Autodesk Inventor part; units mm, degrees
(part 11 of 15)
  arc A4843 (8.9412, 10.184) -> (9.0428, 10.184) centre (8.992, 10.184) ccw
  line L2248 (8.992, 12.216) -> (10.008, 12.216)
  arc A4844 (10.008, 12.1652) -> (10.008, 12.2668) centre (10.008, 12.216) ccw
  arc A4845 (8.992, 12.2668) -> (8.992, 12.1652) centre (8.992, 12.216) ccw
  line L2249 (10.008, 12.216) -> (10.008, 10.184)
  arc A4846 (9.9572, 10.184) -> (10.0588, 10.184) centre (10.008, 10.184) ccw
  arc A4847 (10.0588, 12.216) -> (9.9572, 12.216) centre (10.008, 12.216) ccw
  line L2250 (10.008, 10.184) -> (8.992, 10.184)
  arc A4848 (8.992, 10.2348) -> (8.992, 10.1332) centre (8.992, 10.184) ccw
  arc A4849 (10.008, 10.1332) -> (10.008, 10.2348) centre (10.008, 10.184) ccw
  line L2251 (1.008, 14.216) -> (1.008, 12.184)
  arc A4850 (0.9572, 12.184) -> (1.0588, 12.184) centre (1.008, 12.184) ccw
  arc A4851 (1.0588, 14.216) -> (0.9572, 14.216) centre (1.008, 14.216) ccw
  line L2252 (1.008, 12.184) -> (-0.008, 12.184)
  arc A4852 (-0.008, 12.2348) -> (-0.008, 12.1332) centre (-0.008, 12.184) ccw
  arc A4853 (1.008, 12.1332) -> (1.008, 12.2348) centre (1.008, 12.184) ccw
  line L2253 (-0.008, 12.184) -> (-0.008, 14.216)
  arc A4854 (0.0428, 14.216) -> (-0.0588, 14.216) centre (-0.008, 14.216) ccw
  arc A4855 (-0.0588, 12.184) -> (0.0428, 12.184) centre (-0.008, 12.184) ccw
  line L2254 (-0.008, 14.216) -> (1.008, 14.216)
  arc A4856 (1.008, 14.1652) -> (1.008, 14.2668) centre (1.008, 14.216) ccw
  arc A4857 (-0.008, 14.2668) -> (-0.008, 14.1652) centre (-0.008, 14.216) ccw
  line L2255 (-6.016, 13.208) -> (-3.984, 13.208)
  arc A4858 (-3.984, 13.1572) -> (-3.984, 13.2588) centre (-3.984, 13.208) ccw
  arc A4859 (-6.016, 13.2588) -> (-6.016, 13.1572) centre (-6.016, 13.208) ccw
  line L2256 (-3.984, 13.208) -> (-3.984, 12.192)
  arc A4860 (-4.0348, 12.192) -> (-3.9332, 12.192) centre (-3.984, 12.192) ccw
  arc A4861 (-3.9332, 13.208) -> (-4.0348, 13.208) centre (-3.984, 13.208) ccw
  line L2257 (-3.984, 12.192) -> (-6.016, 12.192)
  arc A4862 (-6.016, 12.2428) -> (-6.016, 12.1412) centre (-6.016, 12.192) ccw
  arc A4863 (-3.984, 12.1412) -> (-3.984, 12.2428) centre (-3.984, 12.192) ccw
  line L2258 (-6.016, 12.192) -> (-6.016, 13.208)
  arc A4864 (-5.9652, 13.208) -> (-6.0668, 13.208) centre (-6.016, 13.208) ccw
  arc A4865 (-6.0668, 12.192) -> (-5.9652, 12.192) centre (-6.016, 12.192) ccw
  line L2259 (-6.016, 12.208) -> (-3.984, 12.208)
  arc A4866 (-3.984, 12.1572) -> (-3.984, 12.2588) centre (-3.984, 12.208) ccw
  arc A4867 (-6.016, 12.2588) -> (-6.016, 12.1572) centre (-6.016, 12.208) ccw
  line L2260 (-3.984, 12.208) -> (-3.984, 11.192)
  arc A4868 (-4.0348, 11.192) -> (-3.9332, 11.192) centre (-3.984, 11.192) ccw
  arc A4869 (-3.9332, 12.208) -> (-4.0348, 12.208) centre (-3.984, 12.208) ccw
  line L2261 (-3.984, 11.192) -> (-6.016, 11.192)
  arc A4870 (-6.016, 11.2428) -> (-6.016, 11.1412) centre (-6.016, 11.192) ccw
  arc A4871 (-3.984, 11.1412) -> (-3.984, 11.2428) centre (-3.984, 11.192) ccw
  line L2262 (-6.016, 11.192) -> (-6.016, 12.208)
  arc A4872 (-5.9652, 12.208) -> (-6.0668, 12.208) centre (-6.016, 12.208) ccw
  arc A4873 (-6.0668, 11.192) -> (-5.9652, 11.192) centre (-6.016, 11.192) ccw
  line L2263 (1.992, -2.816) -> (1.992, -0.784)
  arc A4874 (2.0428, -0.784) -> (1.9412, -0.784) centre (1.992, -0.784) ccw
  arc A4875 (1.9412, -2.816) -> (2.0428, -2.816) centre (1.992, -2.816) ccw
  line L2264 (1.992, -0.784) -> (3.008, -0.784)
  arc A4876 (3.008, -0.8348) -> (3.008, -0.7332) centre (3.008, -0.784) ccw
  arc A4877 (1.992, -0.7332) -> (1.992, -0.8348) centre (1.992, -0.784) ccw
  line L2265 (3.008, -0.784) -> (3.008, -2.816)
  arc A4878 (2.9572, -2.816) -> (3.0588, -2.816) centre (3.008, -2.816) ccw
  arc A4879 (3.0588, -0.784) -> (2.9572, -0.784) centre (3.008, -0.784) ccw
  line L2266 (3.008, -2.816) -> (1.992, -2.816)
  arc A4880 (1.992, -2.7652) -> (1.992, -2.8668) centre (1.992, -2.816) ccw
  arc A4881 (3.008, -2.8668) -> (3.008, -2.7652) centre (3.008, -2.816) ccw
  line L2267 (18.716, 12.192) -> (16.684, 12.192)
  arc A4882 (16.684, 12.2428) -> (16.684, 12.1412) centre (16.684, 12.192) ccw
  arc A4883 (18.716, 12.1412) -> (18.716, 12.2428) centre (18.716, 12.192) ccw
  line L2268 (16.684, 12.192) -> (16.684, 13.208)
  arc A4884 (16.7348, 13.208) -> (16.6332, 13.208) centre (16.684, 13.208) ccw
  arc A4885 (16.6332, 12.192) -> (16.7348, 12.192) centre (16.684, 12.192) ccw
  line L2269 (16.684, 13.208) -> (18.716, 13.208)
  arc A4886 (18.716, 13.1572) -> (18.716, 13.2588) centre (18.716, 13.208) ccw
  arc A4887 (16.684, 13.2588) -> (16.684, 13.1572) centre (16.684, 13.208) ccw
  line L2270 (18.716, 13.208) -> (18.716, 12.192)
  arc A4888 (18.6652, 12.192) -> (18.7668, 12.192) centre (18.716, 12.192) ccw
  arc A4889 (18.7668, 13.208) -> (18.6652, 13.208) centre (18.716, 13.208) ccw
  line L2271 (22.916, 12.192) -> (20.884, 12.192)
  arc A4890 (20.884, 12.2428) -> (20.884, 12.1412) centre (20.884, 12.192) ccw
  arc A4891 (22.916, 12.1412) -> (22.916, 12.2428) centre (22.916, 12.192) ccw
  line L2272 (20.884, 12.192) -> (20.884, 13.208)
  arc A4892 (20.9348, 13.208) -> (20.8332, 13.208) centre (20.884, 13.208) ccw
  arc A4893 (20.8332, 12.192) -> (20.9348, 12.192) centre (20.884, 12.192) ccw
  line L2273 (20.884, 13.208) -> (22.916, 13.208)
  arc A4894 (22.916, 13.1572) -> (22.916, 13.2588) centre (22.916, 13.208) ccw
  arc A4895 (20.884, 13.2588) -> (20.884, 13.1572) centre (20.884, 13.208) ccw
  line L2274 (22.916, 13.208) -> (22.916, 12.192)
  arc A4896 (22.8652, 12.192) -> (22.9668, 12.192) centre (22.916, 12.192) ccw
  arc A4897 (22.9668, 13.208) -> (22.8652, 13.208) centre (22.916, 13.208) ccw
  line L2275 (18.716, 1.792) -> (16.684, 1.792)
  arc A4898 (16.684, 1.8428) -> (16.684, 1.7412) centre (16.684, 1.792) ccw
  arc A4899 (18.716, 1.7412) -> (18.716, 1.8428) centre (18.716, 1.792) ccw
  line L2276 (16.684, 1.792) -> (16.684, 2.808)
  arc A4900 (16.7348, 2.808) -> (16.6332, 2.808) centre (16.684, 2.808) ccw
  arc A4901 (16.6332, 1.792) -> (16.7348, 1.792) centre (16.684, 1.792) ccw
  line L2277 (16.684, 2.808) -> (18.716, 2.808)
  arc A4902 (18.716, 2.7572) -> (18.716, 2.8588) centre (18.716, 2.808) ccw
  arc A4903 (16.684, 2.8588) -> (16.684, 2.7572) centre (16.684, 2.808) ccw
  line L2278 (18.716, 2.808) -> (18.716, 1.792)
  arc A4904 (18.6652, 1.792) -> (18.7668, 1.792) centre (18.716, 1.792) ccw
  arc A4905 (18.7668, 2.808) -> (18.6652, 2.808) centre (18.716, 2.808) ccw
  line L2279 (22.916, 1.792) -> (20.884, 1.792)
  arc A4906 (20.884, 1.8428) -> (20.884, 1.7412) centre (20.884, 1.792) ccw
  arc A4907 (22.916, 1.7412) -> (22.916, 1.8428) centre (22.916, 1.792) ccw
  line L2280 (20.884, 1.792) -> (20.884, 2.808)
  arc A4908 (20.9348, 2.808) -> (20.8332, 2.808) centre (20.884, 2.808) ccw
  arc A4909 (20.8332, 1.792) -> (20.9348, 1.792) centre (20.884, 1.792) ccw
  line L2281 (20.884, 2.808) -> (22.916, 2.808)
  arc A4910 (22.916, 2.7572) -> (22.916, 2.8588) centre (22.916, 2.808) ccw
  arc A4911 (20.884, 2.8588) -> (20.884, 2.7572) centre (20.884, 2.808) ccw
  line L2282 (22.916, 2.808) -> (22.916, 1.792)
  arc A4912 (22.8652, 1.792) -> (22.9668, 1.792) centre (22.916, 1.792) ccw
  arc A4913 (22.9668, 2.808) -> (22.8652, 2.808) centre (22.916, 2.808) ccw
  line L2283 (18.716, -8.608) -> (16.684, -8.608)
  arc A4914 (16.684, -8.5572) -> (16.684, -8.6588) centre (16.684, -8.608) ccw
  arc A4915 (18.716, -8.6588) -> (18.716, -8.5572) centre (18.716, -8.608) ccw
  line L2284 (16.684, -8.608) -> (16.684, -7.592)
  arc A4916 (16.7348, -7.592) -> (16.6332, -7.592) centre (16.684, -7.592) ccw
  arc A4917 (16.6332, -8.608) -> (16.7348, -8.608) centre (16.684, -8.608) ccw
  line L2285 (16.684, -7.592) -> (18.716, -7.592)
  arc A4918 (18.716, -7.6428) -> (18.716, -7.5412) centre (18.716, -7.592) ccw
  arc A4919 (16.684, -7.5412) -> (16.684, -7.6428) centre (16.684, -7.592) ccw
  line L2286 (18.716, -7.592) -> (18.716, -8.608)
  arc A4920 (18.6652, -8.608) -> (18.7668, -8.608) centre (18.716, -8.608) ccw
  arc A4921 (18.7668, -7.592) -> (18.6652, -7.592) centre (18.716, -7.592) ccw
  line L2287 (22.916, -8.608) -> (20.884, -8.608)
  arc A4922 (20.884, -8.5572) -> (20.884, -8.6588) centre (20.884, -8.608) ccw
  arc A4923 (22.916, -8.6588) -> (22.916, -8.5572) centre (22.916, -8.608) ccw
  line L2288 (20.884, -8.608) -> (20.884, -7.592)
  arc A4924 (20.9348, -7.592) -> (20.8332, -7.592) centre (20.884, -7.592) ccw
  arc A4925 (20.8332, -8.608) -> (20.9348, -8.608) centre (20.884, -8.608) ccw
  line L2289 (20.884, -7.592) -> (22.916, -7.592)
  arc A4926 (22.916, -7.6428) -> (22.916, -7.5412) centre (22.916, -7.592) ccw
  arc A4927 (20.884, -7.5412) -> (20.884, -7.6428) centre (20.884, -7.592) ccw
  line L2290 (22.916, -7.592) -> (22.916, -8.608)
  arc A4928 (22.8652, -8.608) -> (22.9668, -8.608) centre (22.916, -8.608) ccw
  arc A4929 (22.9668, -7.592) -> (22.8652, -7.592) centre (22.916, -7.592) ccw
  line L2291 (18.716, -19.008) -> (16.684, -19.008)
  arc A4930 (16.684, -18.9572) -> (16.684, -19.0588) centre (16.684, -19.008) ccw
  arc A4931 (18.716, -19.0588) -> (18.716, -18.9572) centre (18.716, -19.008) ccw
  line L2292 (16.684, -19.008) -> (16.684, -17.992)
  arc A4932 (16.7348, -17.992) -> (16.6332, -17.992) centre (16.684, -17.992) ccw
  arc A4933 (16.6332, -19.008) -> (16.7348, -19.008) centre (16.684, -19.008) ccw
  line L2293 (16.684, -17.992) -> (18.716, -17.992)
  arc A4934 (18.716, -18.0428) -> (18.716, -17.9412) centre (18.716, -17.992) ccw
  arc A4935 (16.684, -17.9412) -> (16.684, -18.0428) centre (16.684, -17.992) ccw
  line L2294 (18.716, -17.992) -> (18.716, -19.008)
  arc A4936 (18.6652, -19.008) -> (18.7668, -19.008) centre (18.716, -19.008) ccw
  arc A4937 (18.7668, -17.992) -> (18.6652, -17.992) centre (18.716, -17.992) ccw
  line L2295 (22.916, -19.008) -> (20.884, -19.008)
  arc A4938 (20.884, -18.9572) -> (20.884, -19.0588) centre (20.884, -19.008) ccw
  arc A4939 (22.916, -19.0588) -> (22.916, -18.9572) centre (22.916, -19.008) ccw
  line L2296 (20.884, -19.008) -> (20.884, -17.992)
  arc A4940 (20.9348, -17.992) -> (20.8332, -17.992) centre (20.884, -17.992) ccw
  arc A4941 (20.8332, -19.008) -> (20.9348, -19.008) centre (20.884, -19.008) ccw
  line L2297 (20.884, -17.992) -> (22.916, -17.992)
  arc A4942 (22.916, -18.0428) -> (22.916, -17.9412) centre (22.916, -17.992) ccw
  arc A4943 (20.884, -17.9412) -> (20.884, -18.0428) centre (20.884, -17.992) ccw
  line L2298 (22.916, -17.992) -> (22.916, -19.008)
  arc A4944 (22.8652, -19.008) -> (22.9668, -19.008) centre (22.916, -19.008) ccw
  arc A4945 (22.9668, -17.992) -> (22.8652, -17.992) centre (22.916, -17.992) ccw
  line L2299 (-1.784, -14.108) -> (-3.816, -14.108)
  arc A4946 (-3.816, -14.0572) -> (-3.816, -14.1588) centre (-3.816, -14.108) ccw
  arc A4947 (-1.784, -14.1588) -> (-1.784, -14.0572) centre (-1.784, -14.108) ccw
  line L2300 (-3.816, -14.108) -> (-3.816, -13.092)
  arc A4948 (-3.7652, -13.092) -> (-3.8668, -13.092) centre (-3.816, -13.092) ccw
  arc A4949 (-3.8668, -14.108) -> (-3.7652, -14.108) centre (-3.816, -14.108) ccw
  line L2301 (-3.816, -13.092) -> (-1.784, -13.092)
  arc A4950 (-1.784, -13.1428) -> (-1.784, -13.0412) centre (-1.784, -13.092) ccw
  arc A4951 (-3.816, -13.0412) -> (-3.816, -13.1428) centre (-3.816, -13.092) ccw
  line L2302 (-1.784, -13.092) -> (-1.784, -14.108)
  arc A4952 (-1.8348, -14.108) -> (-1.7332, -14.108) centre (-1.784, -14.108) ccw
  arc A4953 (-1.7332, -13.092) -> (-1.8348, -13.092) centre (-1.784, -13.092) ccw
  line L2303 (-10.092, -20.084) -> (-10.092, -22.116)
  arc A4954 (-10.1428, -22.116) -> (-10.0412, -22.116) centre (-10.092, -22.116) ccw
  arc A4955 (-10.0412, -20.084) -> (-10.1428, -20.084) centre (-10.092, -20.084) ccw
  line L2304 (-10.092, -22.116) -> (-11.108, -22.116)
  arc A4956 (-11.108, -22.0652) -> (-11.108, -22.1668) centre (-11.108, -22.116) ccw
  arc A4957 (-10.092, -22.1668) -> (-10.092, -22.0652) centre (-10.092, -22.116) ccw
  line L2305 (-11.108, -22.116) -> (-11.108, -20.084)
  arc A4958 (-11.0572, -20.084) -> (-11.1588, -20.084) centre (-11.108, -20.084) ccw
  arc A4959 (-11.1588, -22.116) -> (-11.0572, -22.116) centre (-11.108, -22.116) ccw
  line L2306 (-11.108, -20.084) -> (-10.092, -20.084)
  arc A4960 (-10.092, -20.1348) -> (-10.092, -20.0332) centre (-10.092, -20.084) ccw
  arc A4961 (-11.108, -20.0332) -> (-11.108, -20.1348) centre (-11.108, -20.084) ccw
  line L2307 (-7.216, -23.092) -> (-5.184, -23.092)
  arc A4962 (-5.184, -23.1428) -> (-5.184, -23.0412) centre (-5.184, -23.092) ccw
  arc A4963 (-7.216, -23.0412) -> (-7.216, -23.1428) centre (-7.216, -23.092) ccw
  line L2308 (-5.184, -23.092) -> (-5.184, -24.108)
  arc A4964 (-5.2348, -24.108) -> (-5.1332, -24.108) centre (-5.184, -24.108) ccw
  arc A4965 (-5.1332, -23.092) -> (-5.2348, -23.092) centre (-5.184, -23.092) ccw
  line L2309 (-5.184, -24.108) -> (-7.216, -24.108)
  arc A4966 (-7.216, -24.0572) -> (-7.216, -24.1588) centre (-7.216, -24.108) ccw
  arc A4967 (-5.184, -24.1588) -> (-5.184, -24.0572) centre (-5.184, -24.108) ccw
  line L2310 (-7.216, -24.108) -> (-7.216, -23.092)
  arc A4968 (-7.1652, -23.092) -> (-7.2668, -23.092) centre (-7.216, -23.092) ccw
  arc A4969 (-7.2668, -24.108) -> (-7.1652, -24.108) centre (-7.216, -24.108) ccw
  line L2311 (-1.784, -18.108) -> (-3.816, -18.108)
  arc A4970 (-3.816, -18.0572) -> (-3.816, -18.1588) centre (-3.816, -18.108) ccw
  arc A4971 (-1.784, -18.1588) -> (-1.784, -18.0572) centre (-1.784, -18.108) ccw
  line L2312 (-3.816, -18.108) -> (-3.816, -17.092)
  arc A4972 (-3.7652, -17.092) -> (-3.8668, -17.092) centre (-3.816, -17.092) ccw
  arc A4973 (-3.8668, -18.108) -> (-3.7652, -18.108) centre (-3.816, -18.108) ccw
  line L2313 (-3.816, -17.092) -> (-1.784, -17.092)
  arc A4974 (-1.784, -17.1428) -> (-1.784, -17.0412) centre (-1.784, -17.092) ccw
  arc A4975 (-3.816, -17.0412) -> (-3.816, -17.1428) centre (-3.816, -17.092) ccw
  line L2314 (-1.784, -17.092) -> (-1.784, -18.108)
  arc A4976 (-1.8348, -18.108) -> (-1.7332, -18.108) centre (-1.784, -18.108) ccw
  arc A4977 (-1.7332, -17.092) -> (-1.8348, -17.092) centre (-1.784, -17.092) ccw
  line L2315 (-8.084, -21.108) -> (-10.116, -21.108)
  arc A4978 (-10.116, -21.0572) -> (-10.116, -21.1588) centre (-10.116, -21.108) ccw
  arc A4979 (-8.084, -21.1588) -> (-8.084, -21.0572) centre (-8.084, -21.108) ccw
  line L2316 (-10.116, -21.108) -> (-10.116, -20.092)
  arc A4980 (-10.0652, -20.092) -> (-10.1668, -20.092) centre (-10.116, -20.092) ccw
  arc A4981 (-10.1668, -21.108) -> (-10.0652, -21.108) centre (-10.116, -21.108) ccw
  line L2317 (-10.116, -20.092) -> (-8.084, -20.092)
  arc A4982 (-8.084, -20.1428) -> (-8.084, -20.0412) centre (-8.084, -20.092) ccw
  arc A4983 (-10.116, -20.0412) -> (-10.116, -20.1428) centre (-10.116, -20.092) ccw
  line L2318 (-8.084, -20.092) -> (-8.084, -21.108)
  arc A4984 (-8.1348, -21.108) -> (-8.0332, -21.108) centre (-8.084, -21.108) ccw
  arc A4985 (-8.0332, -20.092) -> (-8.1348, -20.092) centre (-8.084, -20.092) ccw
  line L2319 (-1.784, -20.108) -> (-3.816, -20.108)
  arc A4986 (-3.816, -20.0572) -> (-3.816, -20.1588) centre (-3.816, -20.108) ccw
  arc A4987 (-1.784, -20.1588) -> (-1.784, -20.0572) centre (-1.784, -20.108) ccw
  line L2320 (-3.816, -20.108) -> (-3.816, -19.092)
  arc A4988 (-3.7652, -19.092) -> (-3.8668, -19.092) centre (-3.816, -19.092) ccw
  arc A4989 (-3.8668, -20.108) -> (-3.7652, -20.108) centre (-3.816, -20.108) ccw
  line L2321 (-3.816, -19.092) -> (-1.784, -19.092)
  arc A4990 (-1.784, -19.1428) -> (-1.784, -19.0412) centre (-1.784, -19.092) ccw
  arc A4991 (-3.816, -19.0412) -> (-3.816, -19.1428) centre (-3.816, -19.092) ccw
  line L2322 (-1.784, -19.092) -> (-1.784, -20.108)
  arc A4992 (-1.8348, -20.108) -> (-1.7332, -20.108) centre (-1.784, -20.108) ccw
  arc A4993 (-1.7332, -19.092) -> (-1.8348, -19.092) centre (-1.784, -19.092) ccw
  line L2323 (5.716, -19.808) -> (3.684, -19.808)
  arc A4994 (3.684, -19.7572) -> (3.684, -19.8588) centre (3.684, -19.808) ccw
  arc A4995 (5.716, -19.8588) -> (5.716, -19.7572) centre (5.716, -19.808) ccw
  line L2324 (3.684, -19.808) -> (3.684, -18.792)
  arc A4996 (3.7348, -18.792) -> (3.6332, -18.792) centre (3.684, -18.792) ccw
  arc A4997 (3.6332, -19.808) -> (3.7348, -19.808) centre (3.684, -19.808) ccw
  line L2325 (3.684, -18.792) -> (5.716, -18.792)
  arc A4998 (5.716, -18.8428) -> (5.716, -18.7412) centre (5.716, -18.792) ccw
  arc A4999 (3.684, -18.7412) -> (3.684, -18.8428) centre (3.684, -18.792) ccw
  line L2326 (5.716, -18.792) -> (5.716, -19.808)
  arc A5000 (5.6652, -19.808) -> (5.7668, -19.808) centre (5.716, -19.808) ccw
  arc A5001 (5.7668, -18.792) -> (5.6652, -18.792) centre (5.716, -18.792) ccw
  line L2327 (5.084, -14.792) -> (7.116, -14.792)
  arc A5002 (7.116, -14.8428) -> (7.116, -14.7412) centre (7.116, -14.792) ccw
  arc A5003 (5.084, -14.7412) -> (5.084, -14.8428) centre (5.084, -14.792) ccw
  line L2328 (7.116, -14.792) -> (7.116, -15.808)
  arc A5004 (7.0652, -15.808) -> (7.1668, -15.808) centre (7.116, -15.808) ccw
  arc A5005 (7.1668, -14.792) -> (7.0652, -14.792) centre (7.116, -14.792) ccw
  line L2329 (7.116, -15.808) -> (5.084, -15.808)
  arc A5006 (5.084, -15.7572) -> (5.084, -15.8588) centre (5.084, -15.808) ccw
  arc A5007 (7.116, -15.8588) -> (7.116, -15.7572) centre (7.116, -15.808) ccw
  line L2330 (5.084, -15.808) -> (5.084, -14.792)
  arc A5008 (5.1348, -14.792) -> (5.0332, -14.792) centre (5.084, -14.792) ccw
  arc A5009 (5.0332, -15.808) -> (5.1348, -15.808) centre (5.084, -15.808) ccw
  line L2331 (0.884, -14.792) -> (2.916, -14.792)
  arc A5010 (2.916, -14.8428) -> (2.916, -14.7412) centre (2.916, -14.792) ccw
  arc A5011 (0.884, -14.7412) -> (0.884, -14.8428) centre (0.884, -14.792) ccw
  line L2332 (2.916, -14.792) -> (2.916, -15.808)
  arc A5012 (2.8652, -15.808) -> (2.9668, -15.808) centre (2.916, -15.808) ccw
  arc A5013 (2.9668, -14.792) -> (2.8652, -14.792) centre (2.916, -14.792) ccw
  line L2333 (2.916, -15.808) -> (0.884, -15.808)
  arc A5014 (0.884, -15.7572) -> (0.884, -15.8588) centre (0.884, -15.808) ccw
  arc A5015 (2.916, -15.8588) -> (2.916, -15.7572) centre (2.916, -15.808) ccw
  line L2334 (0.884, -15.808) -> (0.884, -14.792)
  arc A5016 (0.9348, -14.792) -> (0.8332, -14.792) centre (0.884, -14.792) ccw
  arc A5017 (0.8332, -15.808) -> (0.9348, -15.808) centre (0.884, -15.808) ccw
  line L2335 (-7.216, -15.092) -> (-5.184, -15.092)
  arc A5018 (-5.184, -15.1428) -> (-5.184, -15.0412) centre (-5.184, -15.092) ccw
  arc A5019 (-7.216, -15.0412) -> (-7.216, -15.1428) centre (-7.216, -15.092) ccw
  line L2336 (-5.184, -15.092) -> (-5.184, -16.108)
  arc A5020 (-5.2348, -16.108) -> (-5.1332, -16.108) centre (-5.184, -16.108) ccw
  arc A5021 (-5.1332, -15.092) -> (-5.2348, -15.092) centre (-5.184, -15.092) ccw
  line L2337 (-5.184, -16.108) -> (-7.216, -16.108)
  arc A5022 (-7.216, -16.0572) -> (-7.216, -16.1588) centre (-7.216, -16.108) ccw
  arc A5023 (-5.184, -16.1588) -> (-5.184, -16.0572) centre (-5.184, -16.108) ccw
  line L2338 (-7.216, -16.108) -> (-7.216, -15.092)
  arc A5024 (-7.1652, -15.092) -> (-7.2668, -15.092) centre (-7.216, -15.092) ccw
  arc A5025 (-7.2668, -16.108) -> (-7.1652, -16.108) centre (-7.216, -16.108) ccw
  line L2339 (-1.784, -21.108) -> (-3.816, -21.108)
  arc A5026 (-3.816, -21.0572) -> (-3.816, -21.1588) centre (-3.816, -21.108) ccw
  arc A5027 (-1.784, -21.1588) -> (-1.784, -21.0572) centre (-1.784, -21.108) ccw
  line L2340 (-3.816, -21.108) -> (-3.816, -20.092)
  arc A5028 (-3.7652, -20.092) -> (-3.8668, -20.092) centre (-3.816, -20.092) ccw
  arc A5029 (-3.8668, -21.108) -> (-3.7652, -21.108) centre (-3.816, -21.108) ccw
  line L2341 (-3.816, -20.092) -> (-1.784, -20.092)
  arc A5030 (-1.784, -20.1428) -> (-1.784, -20.0412) centre (-1.784, -20.092) ccw
  arc A5031 (-3.816, -20.0412) -> (-3.816, -20.1428) centre (-3.816, -20.092) ccw
  line L2342 (-1.784, -20.092) -> (-1.784, -21.108)
  arc A5032 (-1.8348, -21.108) -> (-1.7332, -21.108) centre (-1.784, -21.108) ccw
  arc A5033 (-1.7332, -20.092) -> (-1.8348, -20.092) centre (-1.784, -20.092) ccw
  line L2343 (-10.116, -23.092) -> (-8.084, -23.092)
  arc A5034 (-8.084, -23.1428) -> (-8.084, -23.0412) centre (-8.084, -23.092) ccw
  arc A5035 (-10.116, -23.0412) -> (-10.116, -23.1428) centre (-10.116, -23.092) ccw
  line L2344 (-8.084, -23.092) -> (-8.084, -24.108)
  arc A5036 (-8.1348, -24.108) -> (-8.0332, -24.108) centre (-8.084, -24.108) ccw
  arc A5037 (-8.0332, -23.092) -> (-8.1348, -23.092) centre (-8.084, -23.092) ccw
  line L2345 (-8.084, -24.108) -> (-10.116, -24.108)
  arc A5038 (-10.116, -24.0572) -> (-10.116, -24.1588) centre (-10.116, -24.108) ccw
  arc A5039 (-8.084, -24.1588) -> (-8.084, -24.0572) centre (-8.084, -24.108) ccw
  line L2346 (-10.116, -24.108) -> (-10.116, -23.092)
  arc A5040 (-10.0652, -23.092) -> (-10.1668, -23.092) centre (-10.116, -23.092) ccw
  arc A5041 (-10.1668, -24.108) -> (-10.0652, -24.108) centre (-10.116, -24.108) ccw
  line L2347 (-1.784, -25.108) -> (-3.816, -25.108)
  arc A5042 (-3.816, -25.0572) -> (-3.816, -25.1588) centre (-3.816, -25.108) ccw
  arc A5043 (-1.784, -25.1588) -> (-1.784, -25.0572) centre (-1.784, -25.108) ccw
  line L2348 (-3.816, -25.108) -> (-3.816, -24.092)
  arc A5044 (-3.7652, -24.092) -> (-3.8668, -24.092) centre (-3.816, -24.092) ccw
  arc A5045 (-3.8668, -25.108) -> (-3.7652, -25.108) centre (-3.816, -25.108) ccw
  line L2349 (-3.816, -24.092) -> (-1.784, -24.092)
  arc A5046 (-1.784, -24.1428) -> (-1.784, -24.0412) centre (-1.784, -24.092) ccw
  arc A5047 (-3.816, -24.0412) -> (-3.816, -24.1428) centre (-3.816, -24.092) ccw
  line L2350 (-1.784, -24.092) -> (-1.784, -25.108)
  arc A5048 (-1.8348, -25.108) -> (-1.7332, -25.108) centre (-1.784, -25.108) ccw
  arc A5049 (-1.7332, -24.092) -> (-1.8348, -24.092) centre (-1.784, -24.092) ccw
  line L2351 (7.892, -20.316) -> (7.892, -18.284)
  arc A5050 (7.9428, -18.284) -> (7.8412, -18.284) centre (7.892, -18.284) ccw
  arc A5051 (7.8412, -20.316) -> (7.9428, -20.316) centre (7.892, -20.316) ccw
  line L2352 (7.892, -18.284) -> (8.908, -18.284)
  arc A5052 (8.908, -18.3348) -> (8.908, -18.2332) centre (8.908, -18.284) ccw
  arc A5053 (7.892, -18.2332) -> (7.892, -18.3348) centre (7.892, -18.284) ccw
  line L2353 (8.908, -18.284) -> (8.908, -20.316)
  arc A5054 (8.8572, -20.316) -> (8.9588, -20.316) centre (8.908, -20.316) ccw
  arc A5055 (8.9588, -18.284) -> (8.8572, -18.284) centre (8.908, -18.284) ccw
  line L2354 (8.908, -20.316) -> (7.892, -20.316)
  arc A5056 (7.892, -20.2652) -> (7.892, -20.3668) centre (7.892, -20.316) ccw
  arc A5057 (8.908, -20.3668) -> (8.908, -20.2652) centre (8.908, -20.316) ccw
  line L2355 (10.892, -20.316) -> (10.892, -18.284)
  arc A5058 (10.9428, -18.284) -> (10.8412, -18.284) centre (10.892, -18.284) ccw
  arc A5059 (10.8412, -20.316) -> (10.9428, -20.316) centre (10.892, -20.316) ccw
  line L2356 (10.892, -18.284) -> (11.908, -18.284)
  arc A5060 (11.908, -18.3348) -> (11.908, -18.2332) centre (11.908, -18.284) ccw
  arc A5061 (10.892, -18.2332) -> (10.892, -18.3348) centre (10.892, -18.284) ccw
  line L2357 (11.908, -18.284) -> (11.908, -20.316)
  arc A5062 (11.8572, -20.316) -> (11.9588, -20.316) centre (11.908, -20.316) ccw
  arc A5063 (11.9588, -18.284) -> (11.8572, -18.284) centre (11.908, -18.284) ccw
  line L2358 (11.908, -20.316) -> (10.892, -20.316)
  arc A5064 (10.892, -20.2652) -> (10.892, -20.3668) centre (10.892, -20.316) ccw
  arc A5065 (11.908, -20.3668) -> (11.908, -20.2652) centre (11.908, -20.316) ccw
  line L2359 (5.684, -18.792) -> (7.716, -18.792)
  arc A5066 (7.716, -18.8428) -> (7.716, -18.7412) centre (7.716, -18.792) ccw
  arc A5067 (5.684, -18.7412) -> (5.684, -18.8428) centre (5.684, -18.792) ccw
  line L2360 (7.716, -18.792) -> (7.716, -19.808)
  arc A5068 (7.6652, -19.808) -> (7.7668, -19.808) centre (7.716, -19.808) ccw
  arc A5069 (7.7668, -18.792) -> (7.6652, -18.792) centre (7.716, -18.792) ccw
  line L2361 (7.716, -19.808) -> (5.684, -19.808)
  arc A5070 (5.684, -19.7572) -> (5.684, -19.8588) centre (5.684, -19.808) ccw
  arc A5071 (7.716, -19.8588) -> (7.716, -19.7572) centre (7.716, -19.808) ccw
  line L2362 (5.684, -19.808) -> (5.684, -18.792)
  arc A5072 (5.7348, -18.792) -> (5.6332, -18.792) centre (5.684, -18.792) ccw
  arc A5073 (5.6332, -19.808) -> (5.7348, -19.808) centre (5.684, -19.808) ccw
  line L2363 (-10.116, -22.092) -> (-8.084, -22.092)
  arc A5074 (-8.084, -22.1428) -> (-8.084, -22.0412) centre (-8.084, -22.092) ccw
  arc A5075 (-10.116, -22.0412) -> (-10.116, -22.1428) centre (-10.116, -22.092) ccw
  line L2364 (-8.084, -22.092) -> (-8.084, -23.108)
  arc A5076 (-8.1348, -23.108) -> (-8.0332, -23.108) centre (-8.084, -23.108) ccw
  arc A5077 (-8.0332, -22.092) -> (-8.1348, -22.092) centre (-8.084, -22.092) ccw
  line L2365 (-8.084, -23.108) -> (-10.116, -23.108)
  arc A5078 (-10.116, -23.0572) -> (-10.116, -23.1588) centre (-10.116, -23.108) ccw
  arc A5079 (-8.084, -23.1588) -> (-8.084, -23.0572) centre (-8.084, -23.108) ccw
  line L2366 (-10.116, -23.108) -> (-10.116, -22.092)
  arc A5080 (-10.0652, -22.092) -> (-10.1668, -22.092) centre (-10.116, -22.092) ccw
  arc A5081 (-10.1668, -23.108) -> (-10.0652, -23.108) centre (-10.116, -23.108) ccw
  line L2367 (-10.116, -21.092) -> (-8.084, -21.092)
  arc A5082 (-8.084, -21.1428) -> (-8.084, -21.0412) centre (-8.084, -21.092) ccw
  arc A5083 (-10.116, -21.0412) -> (-10.116, -21.1428) centre (-10.116, -21.092) ccw
  line L2368 (-8.084, -21.092) -> (-8.084, -22.108)
  arc A5084 (-8.1348, -22.108) -> (-8.0332, -22.108) centre (-8.084, -22.108) ccw
  arc A5085 (-8.0332, -21.092) -> (-8.1348, -21.092) centre (-8.084, -21.092) ccw
  line L2369 (-8.084, -22.108) -> (-10.116, -22.108)
  arc A5086 (-10.116, -22.0572) -> (-10.116, -22.1588) centre (-10.116, -22.108) ccw
  arc A5087 (-8.084, -22.1588) -> (-8.084, -22.0572) centre (-8.084, -22.108) ccw
  line L2370 (-10.116, -22.108) -> (-10.116, -21.092)
  arc A5088 (-10.0652, -21.092) -> (-10.1668, -21.092) centre (-10.116, -21.092) ccw
  arc A5089 (-10.1668, -22.108) -> (-10.0652, -22.108) centre (-10.116, -22.108) ccw
  line L2371 (-19.116, 45.008) -> (-17.084, 45.008)
  arc A5090 (-17.084, 44.9572) -> (-17.084, 45.0588) centre (-17.084, 45.008) ccw
  arc A5091 (-19.116, 45.0588) -> (-19.116, 44.9572) centre (-19.116, 45.008) ccw
  line L2372 (-17.084, 45.008) -> (-17.084, 43.992)
  arc A5092 (-17.1348, 43.992) -> (-17.0332, 43.992) centre (-17.084, 43.992) ccw
  arc A5093 (-17.0332, 45.008) -> (-17.1348, 45.008) centre (-17.084, 45.008) ccw
  line L2373 (-17.084, 43.992) -> (-19.116, 43.992)
  arc A5094 (-19.116, 44.0428) -> (-19.116, 43.9412) centre (-19.116, 43.992) ccw
  arc A5095 (-17.084, 43.9412) -> (-17.084, 44.0428) centre (-17.084, 43.992) ccw
  line L2374 (-19.116, 43.992) -> (-19.116, 45.008)
  arc A5096 (-19.0652, 45.008) -> (-19.1668, 45.008) centre (-19.116, 45.008) ccw
  arc A5097 (-19.1668, 43.992) -> (-19.0652, 43.992) centre (-19.116, 43.992) ccw
  line L2375 (-19.116, 46.008) -> (-17.084, 46.008)
  arc A5098 (-17.084, 45.9572) -> (-17.084, 46.0588) centre (-17.084, 46.008) ccw
  arc A5099 (-19.116, 46.0588) -> (-19.116, 45.9572) centre (-19.116, 46.008) ccw
  line L2376 (-17.084, 46.008) -> (-17.084, 44.992)
  arc A5100 (-17.1348, 44.992) -> (-17.0332, 44.992) centre (-17.084, 44.992) ccw
  arc A5101 (-17.0332, 46.008) -> (-17.1348, 46.008) centre (-17.084, 46.008) ccw
  line L2377 (-17.084, 44.992) -> (-19.116, 44.992)
  arc A5102 (-19.116, 45.0428) -> (-19.116, 44.9412) centre (-19.116, 44.992) ccw
  arc A5103 (-17.084, 44.9412) -> (-17.084, 45.0428) centre (-17.084, 44.992) ccw
  line L2378 (-19.116, 44.992) -> (-19.116, 46.008)
  arc A5104 (-19.0652, 46.008) -> (-19.1668, 46.008) centre (-19.116, 46.008) ccw
  arc A5105 (-19.1668, 44.992) -> (-19.0652, 44.992) centre (-19.116, 44.992) ccw
  line L2379 (-23.284, 38.992) -> (-25.316, 38.992)
  arc A5106 (-25.316, 39.0428) -> (-25.316, 38.9412) centre (-25.316, 38.992) ccw
  arc A5107 (-23.284, 38.9412) -> (-23.284, 39.0428) centre (-23.284, 38.992) ccw
  line L2380 (-25.316, 38.992) -> (-25.316, 40.008)
  arc A5108 (-25.2652, 40.008) -> (-25.3668, 40.008) centre (-25.316, 40.008) ccw
  arc A5109 (-25.3668, 38.992) -> (-25.2652, 38.992) centre (-25.316, 38.992) ccw
  line L2381 (-25.316, 40.008) -> (-23.284, 40.008)
  arc A5110 (-23.284, 39.9572) -> (-23.284, 40.0588) centre (-23.284, 40.008) ccw
  arc A5111 (-25.316, 40.0588) -> (-25.316, 39.9572) centre (-25.316, 40.008) ccw
  line L2382 (-23.284, 40.008) -> (-23.284, 38.992)
  arc A5112 (-23.3348, 38.992) -> (-23.2332, 38.992) centre (-23.284, 38.992) ccw
  arc A5113 (-23.2332, 40.008) -> (-23.3348, 40.008) centre (-23.284, 40.008) ccw
  line L2383 (-22.016, 51.108) -> (-19.984, 51.108)
  arc A5114 (-19.984, 51.0572) -> (-19.984, 51.1588) centre (-19.984, 51.108) ccw
  arc A5115 (-22.016, 51.1588) -> (-22.016, 51.0572) centre (-22.016, 51.108) ccw
  line L2384 (-19.984, 51.108) -> (-19.984, 50.092)
  arc A5116 (-20.0348, 50.092) -> (-19.9332, 50.092) centre (-19.984, 50.092) ccw
  arc A5117 (-19.9332, 51.108) -> (-20.0348, 51.108) centre (-19.984, 51.108) ccw
  line L2385 (-19.984, 50.092) -> (-22.016, 50.092)
  arc A5118 (-22.016, 50.1428) -> (-22.016, 50.0412) centre (-22.016, 50.092) ccw
  arc A5119 (-19.984, 50.0412) -> (-19.984, 50.1428) centre (-19.984, 50.092) ccw
  line L2386 (-22.016, 50.092) -> (-22.016, 51.108)
  arc A5120 (-21.9652, 51.108) -> (-22.0668, 51.108) centre (-22.016, 51.108) ccw
  arc A5121 (-22.0668, 50.092) -> (-21.9652, 50.092) centre (-22.016, 50.092) ccw
  line L2387 (-19.984, 48.092) -> (-22.016, 48.092)
  arc A5122 (-22.016, 48.1428) -> (-22.016, 48.0412) centre (-22.016, 48.092) ccw
  arc A5123 (-19.984, 48.0412) -> (-19.984, 48.1428) centre (-19.984, 48.092) ccw
  line L2388 (-22.016, 48.092) -> (-22.016, 49.108)
  arc A5124 (-21.9652, 49.108) -> (-22.0668, 49.108) centre (-22.016, 49.108) ccw
  arc A5125 (-22.0668, 48.092) -> (-21.9652, 48.092) centre (-22.016, 48.092) ccw
  line L2389 (-22.016, 49.108) -> (-19.984, 49.108)
  arc A5126 (-19.984, 49.0572) -> (-19.984, 49.1588) centre (-19.984, 49.108) ccw
  arc A5127 (-22.016, 49.1588) -> (-22.016, 49.0572) centre (-22.016, 49.108) ccw
  line L2390 (-19.984, 49.108) -> (-19.984, 48.092)
  arc A5128 (-20.0348, 48.092) -> (-19.9332, 48.092) centre (-19.984, 48.092) ccw
  arc A5129 (-19.9332, 49.108) -> (-20.0348, 49.108) centre (-19.984, 49.108) ccw
  line L2391 (-23.292, 42.016) -> (-23.292, 39.984)
  arc A5130 (-23.3428, 39.984) -> (-23.2412, 39.984) centre (-23.292, 39.984) ccw
  arc A5131 (-23.2412, 42.016) -> (-23.3428, 42.016) centre (-23.292, 42.016) ccw
  line L2392 (-23.292, 39.984) -> (-24.308, 39.984)
  arc A5132 (-24.308, 40.0348) -> (-24.308, 39.9332) centre (-24.308, 39.984) ccw
  arc A5133 (-23.292, 39.9332) -> (-23.292, 40.0348) centre (-23.292, 39.984) ccw
  line L2393 (-24.308, 39.984) -> (-24.308, 42.016)
  arc A5134 (-24.2572, 42.016) -> (-24.3588, 42.016) centre (-24.308, 42.016) ccw
  arc A5135 (-24.3588, 39.984) -> (-24.2572, 39.984) centre (-24.308, 39.984) ccw
  line L2394 (-24.308, 42.016) -> (-23.292, 42.016)
  arc A5136 (-23.292, 41.9652) -> (-23.292, 42.0668) centre (-23.292, 42.016) ccw
  arc A5137 (-24.308, 42.0668) -> (-24.308, 41.9652) centre (-24.308, 42.016) ccw
  line L2395 (-20.292, 40.016) -> (-20.292, 37.984)
  arc A5138 (-20.3428, 37.984) -> (-20.2412, 37.984) centre (-20.292, 37.984) ccw
  arc A5139 (-20.2412, 40.016) -> (-20.3428, 40.016) centre (-20.292, 40.016) ccw
  line L2396 (-20.292, 37.984) -> (-21.308, 37.984)
  arc A5140 (-21.308, 38.0348) -> (-21.308, 37.9332) centre (-21.308, 37.984) ccw
  arc A5141 (-20.292, 37.9332) -> (-20.292, 38.0348) centre (-20.292, 37.984) ccw
  line L2397 (-21.308, 37.984) -> (-21.308, 40.016)
  arc A5142 (-21.2572, 40.016) -> (-21.3588, 40.016) centre (-21.308, 40.016) ccw
  arc A5143 (-21.3588, 37.984) -> (-21.2572, 37.984) centre (-21.308, 37.984) ccw
  line L2398 (-21.308, 40.016) -> (-20.292, 40.016)
  arc A5144 (-20.292, 39.9652) -> (-20.292, 40.0668) centre (-20.292, 40.016) ccw
  arc A5145 (-21.308, 40.0668) -> (-21.308, 39.9652) centre (-21.308, 40.016) ccw
  line L2399 (-26.016, 51.108) -> (-23.984, 51.108)
  arc A5146 (-23.984, 51.0572) -> (-23.984, 51.1588) centre (-23.984, 51.108) ccw
  arc A5147 (-26.016, 51.1588) -> (-26.016, 51.0572) centre (-26.016, 51.108) ccw
  line L2400 (-23.984, 51.108) -> (-23.984, 50.092)
  arc A5148 (-24.0348, 50.092) -> (-23.9332, 50.092) centre (-23.984, 50.092) ccw
  arc A5149 (-23.9332, 51.108) -> (-24.0348, 51.108) centre (-23.984, 51.108) ccw
  line L2401 (-23.984, 50.092) -> (-26.016, 50.092)
  arc A5150 (-26.016, 50.1428) -> (-26.016, 50.0412) centre (-26.016, 50.092) ccw
  arc A5151 (-23.984, 50.0412) -> (-23.984, 50.1428) centre (-23.984, 50.092) ccw
  line L2402 (-26.016, 50.092) -> (-26.016, 51.108)
  arc A5152 (-25.9652, 51.108) -> (-26.0668, 51.108) centre (-26.016, 51.108) ccw
  arc A5153 (-26.0668, 50.092) -> (-25.9652, 50.092) centre (-26.016, 50.092) ccw
  line L2403 (-23.984, 46.092) -> (-26.016, 46.092)
  arc A5154 (-26.016, 46.1428) -> (-26.016, 46.0412) centre (-26.016, 46.092) ccw
  arc A5155 (-23.984, 46.0412) -> (-23.984, 46.1428) centre (-23.984, 46.092) ccw
  line L2404 (-26.016, 46.092) -> (-26.016, 47.108)
  arc A5156 (-25.9652, 47.108) -> (-26.0668, 47.108) centre (-26.016, 47.108) ccw
  arc A5157 (-26.0668, 46.092) -> (-25.9652, 46.092) centre (-26.016, 46.092) ccw
  line L2405 (-26.016, 47.108) -> (-23.984, 47.108)
  arc A5158 (-23.984, 47.0572) -> (-23.984, 47.1588) centre (-23.984, 47.108) ccw
  arc A5159 (-26.016, 47.1588) -> (-26.016, 47.0572) centre (-26.016, 47.108) ccw
  line L2406 (-23.984, 47.108) -> (-23.984, 46.092)
  arc A5160 (-24.0348, 46.092) -> (-23.9332, 46.092) centre (-23.984, 46.092) ccw
  arc A5161 (-23.9332, 47.108) -> (-24.0348, 47.108) centre (-23.984, 47.108) ccw
  line L2407 (-23.984, 44.092) -> (-26.016, 44.092)
  arc A5162 (-26.016, 44.1428) -> (-26.016, 44.0412) centre (-26.016, 44.092) ccw
  arc A5163 (-23.984, 44.0412) -> (-23.984, 44.1428) centre (-23.984, 44.092) ccw
  line L2408 (-26.016, 44.092) -> (-26.016, 45.108)
  arc A5164 (-25.9652, 45.108) -> (-26.0668, 45.108) centre (-26.016, 45.108) ccw
  arc A5165 (-26.0668, 44.092) -> (-25.9652, 44.092) centre (-26.016, 44.092) ccw
  line L2409 (-26.016, 45.108) -> (-23.984, 45.108)
  arc A5166 (-23.984, 45.0572) -> (-23.984, 45.1588) centre (-23.984, 45.108) ccw
  arc A5167 (-26.016, 45.1588) -> (-26.016, 45.0572) centre (-26.016, 45.108) ccw
  line L2410 (-23.984, 45.108) -> (-23.984, 44.092)
  arc A5168 (-24.0348, 44.092) -> (-23.9332, 44.092) centre (-23.984, 44.092) ccw
  arc A5169 (-23.9332, 45.108) -> (-24.0348, 45.108) centre (-23.984, 45.108) ccw
  line L2411 (-19.116, 47.008) -> (-17.084, 47.008)
  arc A5170 (-17.084, 46.9572) -> (-17.084, 47.0588) centre (-17.084, 47.008) ccw
  arc A5171 (-19.116, 47.0588) -> (-19.116, 46.9572) centre (-19.116, 47.008) ccw
  line L2412 (-17.084, 47.008) -> (-17.084, 45.992)
  arc A5172 (-17.1348, 45.992) -> (-17.0332, 45.992) centre (-17.084, 45.992) ccw
  arc A5173 (-17.0332, 47.008) -> (-17.1348, 47.008) centre (-17.084, 47.008) ccw
  line L2413 (-17.084, 45.992) -> (-19.116, 45.992)
  arc A5174 (-19.116, 46.0428) -> (-19.116, 45.9412) centre (-19.116, 45.992) ccw
  arc A5175 (-17.084, 45.9412) -> (-17.084, 46.0428) centre (-17.084, 45.992) ccw
  line L2414 (-19.116, 45.992) -> (-19.116, 47.008)
  arc A5176 (-19.0652, 47.008) -> (-19.1668, 47.008) centre (-19.116, 47.008) ccw
  arc A5177 (-19.1668, 45.992) -> (-19.0652, 45.992) centre (-19.116, 45.992) ccw
  line L2415 (-19.116, 48.008) -> (-17.084, 48.008)
  arc A5178 (-17.084, 47.9572) -> (-17.084, 48.0588) centre (-17.084, 48.008) ccw
  arc A5179 (-19.116, 48.0588) -> (-19.116, 47.9572) centre (-19.116, 48.008) ccw
  line L2416 (-17.084, 48.008) -> (-17.084, 46.992)
  arc A5180 (-17.1348, 46.992) -> (-17.0332, 46.992) centre (-17.084, 46.992) ccw
  arc A5181 (-17.0332, 48.008) -> (-17.1348, 48.008) centre (-17.084, 48.008) ccw
  line L2417 (-17.084, 46.992) -> (-19.116, 46.992)
  arc A5182 (-19.116, 47.0428) -> (-19.116, 46.9412) centre (-19.116, 46.992) ccw
  arc A5183 (-17.084, 46.9412) -> (-17.084, 47.0428) centre (-17.084, 46.992) ccw
  line L2418 (-19.116, 46.992) -> (-19.116, 48.008)
  arc A5184 (-19.0652, 48.008) -> (-19.1668, 48.008) centre (-19.116, 48.008) ccw
  arc A5185 (-19.1668, 46.992) -> (-19.0652, 46.992) centre (-19.116, 46.992) ccw
  line L2419 (-49.735, -37.497) -> (-49.735, -34.703)
  arc A5186 (-49.6842, -34.703) -> (-49.7858, -34.703) centre (-49.735, -34.703) ccw
  arc A5187 (-49.7858, -37.497) -> (-49.6842, -37.497) centre (-49.735, -37.497) ccw
  line L2420 (-49.735, -34.703) -> (-48.465, -34.703)
  arc A5188 (-48.465, -34.7538) -> (-48.465, -34.6522) centre (-48.465, -34.703) ccw
  arc A5189 (-49.735, -34.6522) -> (-49.735, -34.7538) centre (-49.735, -34.703) ccw
  line L2421 (-48.465, -34.703) -> (-48.465, -37.497)
  arc A5190 (-48.5158, -37.497) -> (-48.4142, -37.497) centre (-48.465, -37.497) ccw
  arc A5191 (-48.4142, -34.703) -> (-48.5158, -34.703) centre (-48.465, -34.703) ccw
  line L2422 (-48.465, -37.497) -> (-49.735, -37.497)
  arc A5192 (-49.735, -37.4462) -> (-49.735, -37.5478) centre (-49.735, -37.497) ccw
  arc A5193 (-48.465, -37.5478) -> (-48.465, -37.4462) centre (-48.465, -37.497) ccw
  line L2423 (12.5542, -39.989) -> (8.8458, -39.989)
  arc A5194 (8.8458, -39.9382) -> (8.8458, -40.0398) centre (8.8458, -39.989) ccw
  arc A5195 (12.5542, -40.0398) -> (12.5542, -39.9382) centre (12.5542, -39.989) ccw
  line L2424 (8.8458, -39.989) -> (8.8458, -38.211)
  arc A5196 (8.8966, -38.211) -> (8.795, -38.211) centre (8.8458, -38.211) ccw
  arc A5197 (8.795, -39.989) -> (8.8966, -39.989) centre (8.8458, -39.989) ccw
  line L2425 (8.8458, -38.211) -> (12.5542, -38.211)
  arc A5198 (12.5542, -38.2618) -> (12.5542, -38.1602) centre (12.5542, -38.211) ccw
  arc A5199 (8.8458, -38.1602) -> (8.8458, -38.2618) centre (8.8458, -38.211) ccw
  line L2426 (12.5542, -38.211) -> (12.5542, -39.989)
  arc A5200 (12.5034, -39.989) -> (12.605, -39.989) centre (12.5542, -39.989) ccw
  arc A5201 (12.605, -38.211) -> (12.5034, -38.211) centre (12.5542, -38.211) ccw
  line L2427 (12.5542, -41.789) -> (8.8458, -41.789)
  arc A5202 (8.8458, -41.7382) -> (8.8458, -41.8398) centre (8.8458, -41.789) ccw
  arc A5203 (12.5542, -41.8398) -> (12.5542, -41.7382) centre (12.5542, -41.789) ccw
  line L2428 (8.8458, -41.789) -> (8.8458, -40.011)
  arc A5204 (8.8966, -40.011) -> (8.795, -40.011) centre (8.8458, -40.011) ccw
  arc A5205 (8.795, -41.789) -> (8.8966, -41.789) centre (8.8458, -41.789) ccw
  line L2429 (8.8458, -40.011) -> (12.5542, -40.011)
  arc A5206 (12.5542, -40.0618) -> (12.5542, -39.9602) centre (12.5542, -40.011) ccw
  arc A5207 (8.8458, -39.9602) -> (8.8458, -40.0618) centre (8.8458, -40.011) ccw
  line L2430 (12.5542, -40.011) -> (12.5542, -41.789)
  arc A5208 (12.5034, -41.789) -> (12.605, -41.789) centre (12.5542, -41.789) ccw
  arc A5209 (12.605, -40.011) -> (12.5034, -40.011) centre (12.5542, -40.011) ccw
  line L2431 (2.584, -42.592) -> (4.616, -42.592)
  arc A5210 (4.616, -42.6428) -> (4.616, -42.5412) centre (4.616, -42.592) ccw
  arc A5211 (2.584, -42.5412) -> (2.584, -42.6428) centre (2.584, -42.592) ccw
  line L2432 (4.616, -42.592) -> (4.616, -43.608)
  arc A5212 (4.5652, -43.608) -> (4.6668, -43.608) centre (4.616, -43.608) ccw
  arc A5213 (4.6668, -42.592) -> (4.5652, -42.592) centre (4.616, -42.592) ccw
  line L2433 (4.616, -43.608) -> (2.584, -43.608)
  arc A5214 (2.584, -43.5572) -> (2.584, -43.6588) centre (2.584, -43.608) ccw
  arc A5215 (4.616, -43.6588) -> (4.616, -43.5572) centre (4.616, -43.608) ccw
  line L2434 (2.584, -43.608) -> (2.584, -42.592)
  arc A5216 (2.6348, -42.592) -> (2.5332, -42.592) centre (2.584, -42.592) ccw
  arc A5217 (2.5332, -43.608) -> (2.6348, -43.608) centre (2.584, -43.608) ccw
  line L2435 (-41.0458, -58.989) -> (-44.7542, -58.989)
  arc A5218 (-44.7542, -58.9382) -> (-44.7542, -59.0398) centre (-44.7542, -58.989) ccw
  arc A5219 (-41.0458, -59.0398) -> (-41.0458, -58.9382) centre (-41.0458, -58.989) ccw
  line L2436 (-44.7542, -58.989) -> (-44.7542, -57.211)
  arc A5220 (-44.7034, -57.211) -> (-44.805, -57.211) centre (-44.7542, -57.211) ccw
  arc A5221 (-44.805, -58.989) -> (-44.7034, -58.989) centre (-44.7542, -58.989) ccw
  line L2437 (-44.7542, -57.211) -> (-41.0458, -57.211)
  arc A5222 (-41.0458, -57.2618) -> (-41.0458, -57.1602) centre (-41.0458, -57.211) ccw
  arc A5223 (-44.7542, -57.1602) -> (-44.7542, -57.2618) centre (-44.7542, -57.211) ccw
  line L2438 (-41.0458, -57.211) -> (-41.0458, -58.989)
  arc A5224 (-41.0966, -58.989) -> (-40.995, -58.989) centre (-41.0458, -58.989) ccw
  arc A5225 (-40.995, -57.211) -> (-41.0966, -57.211) centre (-41.0458, -57.211) ccw
  line L2439 (54.634, 52.108) -> (56.666, 52.108)
  arc A5226 (56.666, 52.0572) -> (56.666, 52.1588) centre (56.666, 52.108) ccw
  arc A5227 (54.634, 52.1588) -> (54.634, 52.0572) centre (54.634, 52.108) ccw
  line L2440 (56.666, 52.108) -> (56.666, 51.092)
  arc A5228 (56.6152, 51.092) -> (56.7168, 51.092) centre (56.666, 51.092) ccw
  arc A5229 (56.7168, 52.108) -> (56.6152, 52.108) centre (56.666, 52.108) ccw
  line L2441 (56.666, 51.092) -> (54.634, 51.092)
  arc A5230 (54.634, 51.1428) -> (54.634, 51.0412) centre (54.634, 51.092) ccw
  arc A5231 (56.666, 51.0412) -> (56.666, 51.1428) centre (56.666, 51.092) ccw
  line L2442 (54.634, 51.092) -> (54.634, 52.108)
  arc A5232 (54.6848, 52.108) -> (54.5832, 52.108) centre (54.634, 52.108) ccw
  arc A5233 (54.5832, 51.092) -> (54.6848, 51.092) centre (54.634, 51.092) ccw
  line L2443 (56.666, 52.092) -> (54.634, 52.092)
  arc A5234 (54.634, 52.1428) -> (54.634, 52.0412) centre (54.634, 52.092) ccw
  arc A5235 (56.666, 52.0412) -> (56.666, 52.1428) centre (56.666, 52.092) ccw
  line L2444 (54.634, 52.092) -> (54.634, 53.108)
  arc A5236 (54.6848, 53.108) -> (54.5832, 53.108) centre (54.634, 53.108) ccw
  arc A5237 (54.5832, 52.092) -> (54.6848, 52.092) centre (54.634, 52.092) ccw
  line L2445 (54.634, 53.108) -> (56.666, 53.108)
  arc A5238 (56.666, 53.0572) -> (56.666, 53.1588) centre (56.666, 53.108) ccw
  arc A5239 (54.634, 53.1588) -> (54.634, 53.0572) centre (54.634, 53.108) ccw
  line L2446 (56.666, 53.108) -> (56.666, 52.092)
  arc A5240 (56.6152, 52.092) -> (56.7168, 52.092) centre (56.666, 52.092) ccw
  arc A5241 (56.7168, 53.108) -> (56.6152, 53.108) centre (56.666, 53.108) ccw
  line L2447 (57.658, 49.116) -> (57.658, 47.084)
  arc A5242 (57.6072, 47.084) -> (57.7088, 47.084) centre (57.658, 47.084) ccw
  arc A5243 (57.7088, 49.116) -> (57.6072, 49.116) centre (57.658, 49.116) ccw
  line L2448 (57.658, 47.084) -> (56.642, 47.084)
  arc A5244 (56.642, 47.1348) -> (56.642, 47.0332) centre (56.642, 47.084) ccw
  arc A5245 (57.658, 47.0332) -> (57.658, 47.1348) centre (57.658, 47.084) ccw
  line L2449 (56.642, 47.084) -> (56.642, 49.116)
  arc A5246 (56.6928, 49.116) -> (56.5912, 49.116) centre (56.642, 49.116) ccw
  arc A5247 (56.5912, 47.084) -> (56.6928, 47.084) centre (56.642, 47.084) ccw
  line L2450 (56.642, 49.116) -> (57.658, 49.116)
  arc A5248 (57.658, 49.0652) -> (57.658, 49.1668) centre (57.658, 49.116) ccw
  arc A5249 (56.642, 49.1668) -> (56.642, 49.0652) centre (56.642, 49.116) ccw
  line L2451 (57.634, 49.108) -> (59.666, 49.108)
  arc A5250 (59.666, 49.0572) -> (59.666, 49.1588) centre (59.666, 49.108) ccw
  arc A5251 (57.634, 49.1588) -> (57.634, 49.0572) centre (57.634, 49.108) ccw
  line L2452 (59.666, 49.108) -> (59.666, 48.092)
  arc A5252 (59.6152, 48.092) -> (59.7168, 48.092) centre (59.666, 48.092) ccw
  arc A5253 (59.7168, 49.108) -> (59.6152, 49.108) centre (59.666, 49.108) ccw
  line L2453 (59.666, 48.092) -> (57.634, 48.092)
  arc A5254 (57.634, 48.1428) -> (57.634, 48.0412) centre (57.634, 48.092) ccw
  arc A5255 (59.666, 48.0412) -> (59.666, 48.1428) centre (59.666, 48.092) ccw
  line L2454 (57.634, 48.092) -> (57.634, 49.108)
  arc A5256 (57.6848, 49.108) -> (57.5832, 49.108) centre (57.634, 49.108) ccw
  arc A5257 (57.5832, 48.092) -> (57.6848, 48.092) centre (57.634, 48.092) ccw
  line L2455 (56.634, 52.108) -> (58.666, 52.108)
  arc A5258 (58.666, 52.0572) -> (58.666, 52.1588) centre (58.666, 52.108) ccw
  arc A5259 (56.634, 52.1588) -> (56.634, 52.0572) centre (56.634, 52.108) ccw
  line L2456 (58.666, 52.108) -> (58.666, 51.092)
  arc A5260 (58.6152, 51.092) -> (58.7168, 51.092) centre (58.666, 51.092) ccw
  arc A5261 (58.7168, 52.108) -> (58.6152, 52.108) centre (58.666, 52.108) ccw
  line L2457 (58.666, 51.092) -> (56.634, 51.092)
  arc A5262 (56.634, 51.1428) -> (56.634, 51.0412) centre (56.634, 51.092) ccw
  arc A5263 (58.666, 51.0412) -> (58.666, 51.1428) centre (58.666, 51.092) ccw
  line L2458 (56.634, 51.092) -> (56.634, 52.108)
  arc A5264 (56.6848, 52.108) -> (56.5832, 52.108) centre (56.634, 52.108) ccw
  arc A5265 (56.5832, 51.092) -> (56.6848, 51.092) centre (56.634, 51.092) ccw
  line L2459 (55.642, 49.084) -> (55.642, 51.116)
  arc A5266 (55.6928, 51.116) -> (55.5912, 51.116) centre (55.642, 51.116) ccw
  arc A5267 (55.5912, 49.084) -> (55.6928, 49.084) centre (55.642, 49.084) ccw
  line L2460 (55.642, 51.116) -> (56.658, 51.116)
  arc A5268 (56.658, 51.0652) -> (56.658, 51.1668) centre (56.658, 51.116) ccw
  arc A5269 (55.642, 51.1668) -> (55.642, 51.0652) centre (55.642, 51.116) ccw
  line L2461 (56.658, 51.116) -> (56.658, 49.084)
  arc A5270 (56.6072, 49.084) -> (56.7088, 49.084) centre (56.658, 49.084) ccw
  arc A5271 (56.7088, 51.116) -> (56.6072, 51.116) centre (56.658, 51.116) ccw
  line L2462 (56.658, 49.084) -> (55.642, 49.084)
  arc A5272 (55.642, 49.1348) -> (55.642, 49.0332) centre (55.642, 49.084) ccw
  arc A5273 (56.658, 49.0332) -> (56.658, 49.1348) centre (56.658, 49.084) ccw
  line L2463 (54.658, 51.116) -> (54.658, 49.084)
  arc A5274 (54.6072, 49.084) -> (54.7088, 49.084) centre (54.658, 49.084) ccw
  arc A5275 (54.7088, 51.116) -> (54.6072, 51.116) centre (54.658, 51.116) ccw
  line L2464 (54.658, 49.084) -> (53.642, 49.084)
  arc A5276 (53.642, 49.1348) -> (53.642, 49.0332) centre (53.642, 49.084) ccw
  arc A5277 (54.658, 49.0332) -> (54.658, 49.1348) centre (54.658, 49.084) ccw
  line L2465 (53.642, 49.084) -> (53.642, 51.116)
  arc A5278 (53.6928, 51.116) -> (53.5912, 51.116) centre (53.642, 51.116) ccw
  arc A5279 (53.5912, 49.084) -> (53.6928, 49.084) centre (53.642, 49.084) ccw
  line L2466 (53.642, 51.116) -> (54.658, 51.116)
  arc A5280 (54.658, 51.0652) -> (54.658, 51.1668) centre (54.658, 51.116) ccw
  arc A5281 (53.642, 51.1668) -> (53.642, 51.0652) centre (53.642, 51.116) ccw
  line L2467 (57.642, 49.084) -> (57.642, 51.116)
  arc A5282 (57.6928, 51.116) -> (57.5912, 51.116) centre (57.642, 51.116) ccw
  arc A5283 (57.5912, 49.084) -> (57.6928, 49.084) centre (57.642, 49.084) ccw
  line L2468 (57.642, 51.116) -> (58.658, 51.116)
  arc A5284 (58.658, 51.0652) -> (58.658, 51.1668) centre (58.658, 51.116) ccw
  arc A5285 (57.642, 51.1668) -> (57.642, 51.0652) centre (57.642, 51.116) ccw
  line L2469 (58.658, 51.116) -> (58.658, 49.084)
  arc A5286 (58.6072, 49.084) -> (58.7088, 49.084) centre (58.658, 49.084) ccw
  arc A5287 (58.7088, 51.116) -> (58.6072, 51.116) centre (58.658, 51.116) ccw
  line L2470 (58.658, 49.084) -> (57.642, 49.084)
  arc A5288 (57.642, 49.1348) -> (57.642, 49.0332) centre (57.642, 49.084) ccw
  arc A5289 (58.658, 49.0332) -> (58.658, 49.1348) centre (58.658, 49.084) ccw
  line L2471 (57.658, 51.116) -> (57.658, 49.084)
  arc A5290 (57.6072, 49.084) -> (57.7088, 49.084) centre (57.658, 49.084) ccw
  arc A5291 (57.7088, 51.116) -> (57.6072, 51.116) centre (57.658, 51.116) ccw
  line L2472 (57.658, 49.084) -> (56.642, 49.084)
  arc A5292 (56.642, 49.1348) -> (56.642, 49.0332) centre (56.642, 49.084) ccw
  arc A5293 (57.658, 49.0332) -> (57.658, 49.1348) centre (57.658, 49.084) ccw
  line L2473 (56.642, 49.084) -> (56.642, 51.116)
  arc A5294 (56.6928, 51.116) -> (56.5912, 51.116) centre (56.642, 51.116) ccw
  arc A5295 (56.5912, 49.084) -> (56.6928, 49.084) centre (56.642, 49.084) ccw
  line L2474 (56.642, 51.116) -> (57.658, 51.116)
  arc A5296 (57.658, 51.0652) -> (57.658, 51.1668) centre (57.658, 51.116) ccw
  arc A5297 (56.642, 51.1668) -> (56.642, 51.0652) centre (56.642, 51.116) ccw
  line L2475 (9.616, 50.992) -> (7.584, 50.992)
  arc A5298 (7.584, 51.0428) -> (7.584, 50.9412) centre (7.584, 50.992) ccw
  arc A5299 (9.616, 50.9412) -> (9.616, 51.0428) centre (9.616, 50.992) ccw
  line L2476 (7.584, 50.992) -> (7.584, 52.008)
  arc A5300 (7.6348, 52.008) -> (7.5332, 52.008) centre (7.584, 52.008) ccw
  arc A5301 (7.5332, 50.992) -> (7.6348, 50.992) centre (7.584, 50.992) ccw
  line L2477 (7.584, 52.008) -> (9.616, 52.008)
  arc A5302 (9.616, 51.9572) -> (9.616, 52.0588) centre (9.616, 52.008) ccw
  arc A5303 (7.584, 52.0588) -> (7.584, 51.9572) centre (7.584, 52.008) ccw
  line L2478 (9.616, 52.008) -> (9.616, 50.992)
  arc A5304 (9.5652, 50.992) -> (9.6668, 50.992) centre (9.616, 50.992) ccw
  arc A5305 (9.6668, 52.008) -> (9.5652, 52.008) centre (9.616, 52.008) ccw
  line L2479 (9.616, 51.992) -> (7.584, 51.992)
  arc A5306 (7.584, 52.0428) -> (7.584, 51.9412) centre (7.584, 51.992) ccw
  arc A5307 (9.616, 51.9412) -> (9.616, 52.0428) centre (9.616, 51.992) ccw
  line L2480 (7.584, 51.992) -> (7.584, 53.008)
  arc A5308 (7.6348, 53.008) -> (7.5332, 53.008) centre (7.584, 53.008) ccw
  arc A5309 (7.5332, 51.992) -> (7.6348, 51.992) centre (7.584, 51.992) ccw
  line L2481 (7.584, 53.008) -> (9.616, 53.008)
  arc A5310 (9.616, 52.9572) -> (9.616, 53.0588) centre (9.616, 53.008) ccw
  arc A5311 (7.584, 53.0588) -> (7.584, 52.9572) centre (7.584, 53.008) ccw
  line L2482 (9.616, 53.008) -> (9.616, 51.992)
  arc A5312 (9.5652, 51.992) -> (9.6668, 51.992) centre (9.616, 51.992) ccw